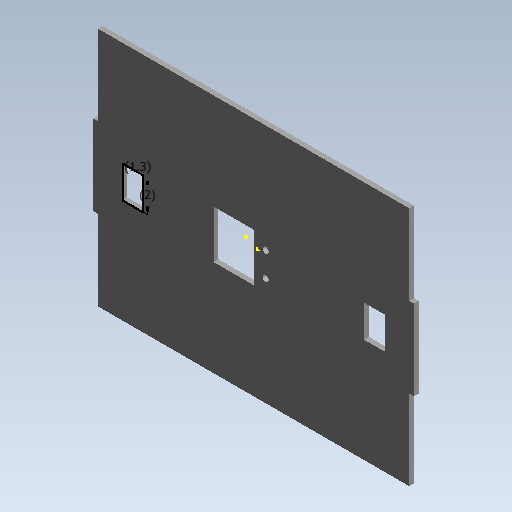
# Autodesk Inventor part: Level1
Saved by Autodesk Inventor 2020 (Build 240168000, 168)
## iProperties
Part Number: Level1
Material: Generic
Document SubType Name: Modeling
Designer: SBBA
Appearance: Default
Mass: 83.9813 g
Surface Area: 587.966 cm^2
Volume: 83.9813 cm^3
Density: 1 g/cm^3
Author: SBBA
Autodesk Inventor part; units mm, degrees
ref_plane "YZ Plane" through (0, 0, 0) normal (1, 0, 0) x (0, 1, 0)
ref_plane "XZ Plane" through (0, 0, 0) normal (0, 1, 0) x (-1, 0, 0)
ref_plane "XY Plane" through (0, 0, 0) normal (0, 0, 1) x (1, 0, 0)
sketch "Sketch1" plane through (0, 0, 0) normal (0, 0, 1) x (1, 0, 0)
  line L0 (-102.5157, 69.2842) -> (97.4843, 69.2842)
  line L1 (97.4843, 69.2842) -> (97.4843, -80.7158)
  line L2 (97.4843, -80.7158) -> (-102.5157, -80.7158)
  line L3 (-102.5157, -80.7158) -> (-102.5157, 69.2842)
  point P0 (0, 0)
  constraints: 8 end point, 2 parallel, 1 horizontal, 1 perpendicular
extrude "Extrusion1" add sketch "Sketch1" along normal blind 3
sketch "Sketch3" plane through (0, 0, 3) normal (0, 0, 1) x (1, 0, 0)
  point P0 (0, 0)
sketch "Sketch4" plane through (0, 0, 3) normal (0, 0, 1) x (1, 0, 0)
  line L0 (97.4843, 69.2842) -> (-102.5157, 69.2842) projected
  line L1 (-102.5157, 69.2842) -> (-99.5157, 69.2842)
  line L2 (-99.5157, 69.2842) -> (-99.5157, 19.2842)
  line L3 (-99.5157, 19.2842) -> (-102.5157, 19.2842)
  line L4 (-102.5157, 19.2842) -> (-102.5157, 69.2842)
  point P0 (0, 0)
  constraints: 8 end point, 2 parallel, 1 horizontal, 1 perpendicular
extrude "Extrusion2" cut sketch "Sketch4" against normal blind 3
sketch "Sketch5" plane through (0, 0, 3) normal (0, 0, 1) x (1, 0, 0)
  line L0 (97.4843, -80.7158) -> (94.4843, -80.7158)
  line L1 (94.4843, -80.7158) -> (94.4843, -30.7158)
  line L2 (94.4843, -30.7158) -> (97.4843, -30.7158)
  line L3 (97.4843, -30.7158) -> (97.4843, -80.7158)
  point P0 (0, 0)
  point P1 (-102.5157, -80.7158)
  dimension "d17" = 3
  dimension "d18" = 50
  constraints: 8 end point, 2 parallel, 1 horizontal, 1 perpendicular
  measures "d17" distance of L1.end L2.end
  measures "d18" distance of L2.end L0.start
extrude "Extrusion3" cut sketch "Sketch5" against normal blind 3
sketch "Sketch6" plane through (0, 0, 3) normal (0, 0, 1) x (1, 0, 0)
  line L0 (97.4843, -30.7158) -> (97.4843, 69.2842) projected
  line L1 (97.4843, 69.2842) -> (94.4843, 69.2842)
  line L2 (94.4843, 69.2842) -> (94.4843, 19.2842)
  line L3 (94.4843, 19.2842) -> (97.4843, 19.2842)
  line L4 (97.4843, 19.2842) -> (97.4843, 69.2842)
  point P0 (0, 0)
  dimension "d21" = 50
  dimension "d22" = 3
  constraints: 8 end point, 2 parallel, 1 horizontal, 1 perpendicular
  measures "d21" distance of L1.end L2.end
  measures "d22" distance of L0.end L1.end
extrude "Extrusion4" cut sketch "Sketch6" against normal blind 3
sketch "Sketch7" plane through (0, 0, 3) normal (0, 0, 1) x (1, 0, 0)
  line L0 (-102.5157, 19.2842) -> (-102.5157, -80.7158) projected
  line L1 (-102.5157, -80.7158) -> (-99.5157, -80.7158)
  line L2 (-99.5157, -80.7158) -> (-99.5157, -30.7158)
  line L3 (-99.5157, -30.7158) -> (-102.5157, -30.7158)
  line L4 (-102.5157, -30.7158) -> (-102.5157, -80.7158)
  point P0 (0, 0)
  dimension "d25" = 50
  dimension "d26" = 3
  constraints: 8 end point, 2 parallel, 1 horizontal, 1 perpendicular
  measures "d25" distance of L1.end L2.end
  measures "d26" distance of L2.end L3.end
extrude "Extrusion5" cut sketch "Sketch7" against normal blind 3
sketch "Sketch8" plane through (0, 0, 3) normal (0, 0, 1) x (1, 0, 0)
  line L0 (-102.5157, -30.7158) -> (-102.5157, 19.2842) projected
  line L1 (97.4843, -30.7158) -> (94.4843, -30.7158) projected
  line L2 (94.4843, -80.7158) -> (-99.5157, -80.7158) projected
  line L3 (-10.0157, -50.7158) -> (4.9843, -50.7158)
  line L4 (4.9843, -50.7158) -> (4.9843, -80.7158)
  line L5 (4.9843, -80.7158) -> (-10.0157, -80.7158)
  line L6 (-10.0157, -80.7158) -> (-10.0157, -50.7158)
  point P0 (0, 0)
  dimension "d32" = 15
  dimension "d33" = 30
  constraints: 8 end point, 2 parallel, 1 horizontal, 1 perpendicular, 1 point on line
  measures "d32" distance of L3.start L3.end
  measures "d33" distance of L3.end L4.end
extrude "Extrusion6" cut sketch "Sketch8" against normal blind 3
sketch "Sketch9" plane through (-10.0157, -80.7158, 3) normal (1, 0, 0) x (0, 0, -1)
  point P0 (3, 80.7158)
sketch "Sketch10" plane through (-10.0157, -50.7158, 3) normal (0, -1, 0) x (1, 0, 0)
  line L0 (15, 0) -> (15, -3) projected
  line L1 (15, -3) -> (0, -3) projected
  line L2 (15, 0) -> (0, 0)
  line L3 (0, 0) -> (0, -3)
  line L4 (0, -3) -> (15, -3)
  line L5 (15, -3) -> (15, 0)
  point P0 (10.0157, -3)
  constraints: 8 end point, 2 parallel, 1 horizontal, 1 perpendicular
extrude "Extrusion7" add sketch "Sketch10" along normal blind 30
sketch "Sketch11" plane through (0, 0, 3) normal (0, 0, 1) x (1, 0, 0)
  line L0 (-102.5157, 19.2842) -> (-99.5157, 19.2842) projected
  line L1 (-99.5157, 69.2842) -> (94.4843, 69.2842) projected
  line L2 (94.4843, -80.7158) -> (-99.5157, -80.7158) projected
  line L3 (-99.5157, 19.2842) -> (-99.5157, 69.2842) projected
  line L4 (-102.5157, -30.7158) -> (-102.5157, 19.2842) projected
  line L5 (-2.5157, 9.2842) -> (-27.5157, 9.2842)
  line L6 (-2.5157, 9.2842) -> (-2.5157, -20.7158)
  line L7 (-27.5157, 9.2842) -> (-27.5157, -20.7158)
  line L8 (-2.5157, -20.7158) -> (-27.5157, -20.7158)
  circle A0 centre (4.9843, 1.9042) radius 2
  circle A1 centre (4.9843, -13.3358) radius 2
  point P0 (0, 0)
  constraints: 8 end point, 2 centre point, 2 horizontal, 2 vertical
extrude "Extrusion8" cut sketch "Sketch11" against normal blind 21.5
sketch "Sketch12" plane through (0, 0, 3) normal (0, 0, 1) x (1, 0, 0)
  point P0 (0, 0)
sketch "Sketch13" plane through (0, 0, 3) normal (0, 0, 1) x (1, 0, 0)
  point P0 (0, 0)
sketch "Sketch14" plane through (0, 0, 3) normal (0, 0, 1) x (1, 0, 0)
  line L0 (97.4843, 19.2842) -> (97.4843, -30.7158) projected
  line L1 (-2.5157, -20.7158) -> (-2.5157, 9.2842) projected
  line L2 (36.2282, 8.4721) -> (58.5282, 8.4721)
  line L3 (58.5282, 8.4721) -> (58.5282, -19.8279)
  line L4 (58.5282, -19.8279) -> (36.2282, -19.8279)
  line L5 (36.2282, -19.8279) -> (36.2282, 8.4721)
  line L6 (-99.5157, 69.2842) -> (94.4843, 69.2842) projected
  point P0 (0, 0)
  constraints: 8 end point, 2 parallel, 1 horizontal, 1 perpendicular
extrude "Extrusion9" cut sketch "Sketch14" against normal blind 30
sketch "Sketch15" plane through (0, 0, 3) normal (0, 0, 1) x (1, 0, 0)
  line L0 (36.2282, -19.8279) -> (36.2282, 8.4721) projected
  line L1 (36.2282, -19.8279) -> (58.5282, -19.8279) projected
  line L2 (36.2282, 8.4721) -> (58.5282, 8.4721)
  line L3 (58.5282, 8.4721) -> (58.5282, -19.8279)
  line L4 (58.5282, -19.8279) -> (36.2282, -19.8279)
  line L5 (36.2282, -19.8279) -> (36.2282, 8.4721)
  point P0 (0, 0)
  constraints: 8 end point, 2 parallel, 1 horizontal, 1 perpendicular
extrude "Extrusion10" add sketch "Sketch15" against normal blind 3
sketch "Sketch16" plane through (0, 0, 3) normal (0, 0, 1) x (1, 0, 0)
  line L0 (-102.5157, -30.7158) -> (-102.5157, 19.2842) projected
  line L1 (97.4843, 19.2842) -> (97.4843, -30.7158) projected
  line L2 (-99.5157, 69.2842) -> (94.4843, 69.2842) projected
  line L3 (40.9489, 4.2992) -> (53.9459, 4.2992)
  line L4 (53.9459, 4.2992) -> (53.9459, -15.7008)
  line L5 (53.9459, -15.7008) -> (40.9489, -15.7008)
  line L6 (40.9489, -15.7008) -> (40.9489, 4.2992)
  point P0 (0, 0)
  constraints: 8 end point, 2 parallel, 1 horizontal, 1 perpendicular
extrude "Extrusion11" cut sketch "Sketch16" against normal blind 3
sketch "Sketch17" plane through (0, 0, 3) normal (0, 0, 1) x (1, 0, 0)
  line L0 (40.9489, -15.7008) -> (40.9489, 4.2992) projected
  line L1 (-102.5157, -30.7158) -> (-102.5157, 19.2842) projected
  line L2 (53.9459, -15.7008) -> (53.9459, 4.2992) projected
  line L3 (97.4843, 19.2842) -> (97.4843, -30.7158) projected
  line L4 (40.9489, 4.2992) -> (53.9459, 4.2992)
  line L5 (53.9459, 4.2992) -> (53.9459, -15.7008)
  line L6 (53.9459, -15.7008) -> (40.9489, -15.7008)
  line L7 (40.9489, -15.7008) -> (40.9489, 4.2992)
  point P0 (0, 0)
  constraints: 8 end point, 2 parallel, 1 horizontal, 1 perpendicular
extrude "Extrusion12" add sketch "Sketch17" against normal blind 3
sketch "Sketch18" plane through (0, 0, 3) normal (0, 0, 1) x (1, 0, 0)
  line L0 (97.4843, 19.2842) -> (97.4843, -30.7158) projected
  line L1 (-102.5157, -30.7158) -> (-102.5157, 19.2842) projected
  line L2 (-84.5157, 4.2842) -> (-71.5157, 4.2842)
  line L3 (-84.5157, 4.2842) -> (-71.5157, 4.2842)
  line L4 (-71.5157, 4.2842) -> (-71.5157, -15.7158)
  line L5 (-71.5157, -15.7158) -> (-84.5157, -15.7158)
  line L6 (-84.5157, -15.7158) -> (-84.5157, 4.2842)
  line L7 (79.4843, 4.2842) -> (66.4843, 4.2842)
  line L8 (79.4843, 4.2842) -> (66.4843, 4.2842)
  line L9 (66.4843, 4.2842) -> (66.4843, -15.7158)
  line L10 (66.4843, -15.7158) -> (79.4843, -15.7158)
  line L11 (79.4843, -15.7158) -> (79.4843, 4.2842)
  point P0 (0, 0)
  constraints: 20 end point, 4 horizontal, 4 parallel, 2 perpendicular
extrude "Extrusion13" cut sketch "Sketch18" against normal blind 3
sketch "Sketch19" plane through (0, 0, 3) normal (0, 0, 1) x (1, 0, 0)
  point P0 (0, 0)
sketch "Sketch20" plane through (0, 0, 3) normal (0, 0, 1) x (1, 0, 0)
  line L0 (-84.5157, 4.2842) -> (-84.5157, -15.7158) projected
  line L1 (-71.5157, -15.7158) -> (-71.5157, 4.2842) projected
  line L2 (-84.5157, 4.2842) -> (-71.5157, 4.2842)
  line L3 (-71.5157, 4.2842) -> (-71.5157, -15.7158)
  line L4 (-71.5157, -15.7158) -> (-84.5157, -15.7158)
  line L5 (-84.5157, -15.7158) -> (-84.5157, 4.2842)
  point P0 (0, 0)
  dimension "d102" = 13
  dimension "d103" = 20
  constraints: 8 end point, 2 parallel, 1 horizontal, 1 perpendicular
  measures "d102" distance of L0.start L2.end
  measures "d103" distance of L1.start L1.end
body "Solid1"
